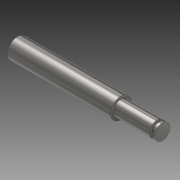
# Autodesk Inventor part: thumb_opposing_worm_shaft
Saved by Autodesk Inventor 2017 SP1 (Build 210196100, 196)
## iProperties
Created: 2017-07-12
Part Number: thumb_opposing_worm_shaft
Material: Stainless Steel
Document SubType Name: Modeling
Designer: JT
Density: 8 g/cm^3
Appearance: Semi-Polished
Author: JT
Autodesk Inventor part; units mm, degrees
ref_plane "YZ Plane" through (0, 0, 0) normal (1, 0, 0) x (0, 1, 0)
ref_plane "XZ Plane" through (0, 0, 0) normal (0, 1, 0) x (-1, 0, 0)
ref_plane "XY Plane" through (0, 0, 0) normal (0, 0, 1) x (1, 0, 0)
sketch "Sketch1" plane through (0, 0, 0) normal (0, 0, 1) x (1, 0, 0)
  line L0 (0, 0) -> (0, 2)
  line L1 (0, 2) -> (20.2, 2)
  line L2 (20.2, 2) -> (20.2, 1.5)
  line L3 (20.2, 1.5) -> (27.3, 1.5)
  line L4 (27.3, 1.5) -> (27.3, 1)
  line L5 (27.3, 1) -> (27.8, 1)
  line L6 (27.8, 1) -> (27.8, 1.5)
  line L7 (27.8, 1.5) -> (28.3, 1.5)
  line L8 (28.3, 1.5) -> (28.3, 0)
  line L9 (28.3, 0) -> (0, 0)
  dimension "d0" = 4
  dimension "d1" = 3
  dimension "d2" = 0.5
  dimension "d3" = 0.5
  dimension "d4" = 0.5
  dimension "d5" = 7.1
  dimension "d6" = 20.2
  constraints: 20 end point, 8 perpendicular, 2 point on line, 1 vertical
  measures "d0" diameter of L1 L9
  measures "d1" diameter of L3 L9
  measures "d2" distance between parallel lines of L6 L4
  measures "d3" distance between parallel lines of L7 L5
  measures "d4" distance between parallel lines of L8 L6
  measures "d5" distance between parallel lines of L4 L2
  measures "d6" distance from line of L0 L2.end
revolve "Revolution1" add sketch "Sketch1" angle 360 about axis through (28.3, 0, 0) along (-1, 0, 0)
hole "Hole1" at (0, 0, 0) direction (1, 0, 0) diameter 3 depth 6 tip angle 118
body "Solid1"
